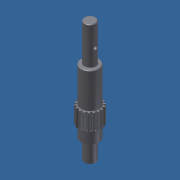
# Autodesk Inventor part: ENGR.HELICOIDAL MOTORA(20)
Saved by Autodesk Inventor 2012 SP2 (Build 160219200, 219)
## iProperties
Created: 2012-07-24
Part Number: ENGR.HELICOIDAL MOTORA(20)
Material: Carbon Steel
Document SubType Name: Modeling
Designer: bruno.silveira
Mass: 284.519 g
Surface Area: 75.4255 cm^2
Volume: 36.1524 cm^3
Density: 7.87 g/cm^3
Author: bruno.silveira
Autodesk Inventor part; units mm, degrees
ref_plane "YZ Plane" through (0, 0, 0) normal (1, 0, 0) x (0, 1, 0)
ref_plane "XZ Plane" through (0, 0, 0) normal (0, 1, 0) x (-1, 0, 0)
ref_plane "XY Plane" through (0, 0, 0) normal (0, 0, 1) x (1, 0, 0)
sketch "Sketch1" plane through (0, 0, 0) normal (0, 0, 1) x (1, 0, 0)
  circle A0 centre (0, 0) radius 10.57
  dimension "d0" = 21.14
  constraints: 1 centre point, 1 coincident
  measures "d0" diameter of A0
extrude "Extrusion1" add sketch "Sketch1" along normal blind 108
sketch "Sketch2" plane through (0, 0, 108) normal (0, 0, 1) x (1, 0, 0)
  circle A0 centre (0, 0) radius 10.57 projected
  circle A1 centre (0, 0) radius 5
  dimension "d3" = 10
  constraints: 1 centre point, 1 coincident
  measures "d3" diameter of A1
extrude "Extrusion2" cut sketch "Sketch2" against normal blind 33.5
sketch "Sketch3" plane through (0, 0, 108) normal (0, 0, 1) x (1, 0, 0)
  circle A0 centre (0, 0) radius 5 projected
  circle A1 centre (0, 0) radius 8
  circle A2 centre (0, 0) radius 10.57 projected
  dimension "d6" = 16
  constraints: 1 centre point, 1 coincident
  measures "d6" diameter of A1
extrude "Extrusion3" cut sketch "Sketch3" against normal blind 65 contours A2
sketch "Sketch4" plane through (0, 0, 0) normal (0, 0, -1) x (-1, 0, 0)
  circle A0 centre (0, 0) radius 10.57 projected
  circle A1 centre (0, 0) radius 5
  dimension "d9" = 10
  constraints: 1 centre point, 1 coincident
  measures "d9" diameter of A1
extrude "Extrusion4" cut sketch "Sketch4" against normal blind 17
sketch "Sketch5" plane through (0, 0, 17) normal (0, 0, -1) x (-1, 0, 0)
  circle A0 centre (0, 0) radius 10.57 projected
  circle A1 centre (0, 0) radius 8
  dimension "d12" = 16
  constraints: 1 centre point, 1 coincident
  measures "d12" diameter of A1
extrude "Extrusion5" cut sketch "Sketch5" against normal blind 11
chamfer "Chamfer1" distance 0.5 angle 45 4 edges at (5, 0, 0) (-5, 0, 108) (8, 0, 17) (-8, 0, 74.5)
fillet "Fillet1" radius 0.5 4 edges at (-5, 0, 74.5) (-8, 0, 43) (8, 0, 28) (5, 0, 17)
spur gear teeth "Spur Gear1" teeth 18 pitch diameter 19.1552 tip diameter 21.1546 root diameter 16.6552 face width 15 helix angle 20 hand right trims to tip circle yes start plane through (0, 0, 28) normal (0, 0, -1) x (-1, 0, 0)
sketch "Sketch6" plane through (0, 0, 0) normal (1, 0, 0) x (0, 1, 0)
  circle A0 centre (0, 89) radius 1.5
  line L0 (-4.5, 108) -> (4.5, 108) projected
  point P0 (0, 0)
  dimension "d19" = 3
  dimension "d20" = 19
  constraints: 1 centre point
  measures "d19" diameter of A0
  measures "d20" distance from line of L0 A0.centre
extrude "Extrusion6" cut sketch "Sketch6" along normal mid plane 12
body "Solid1"
